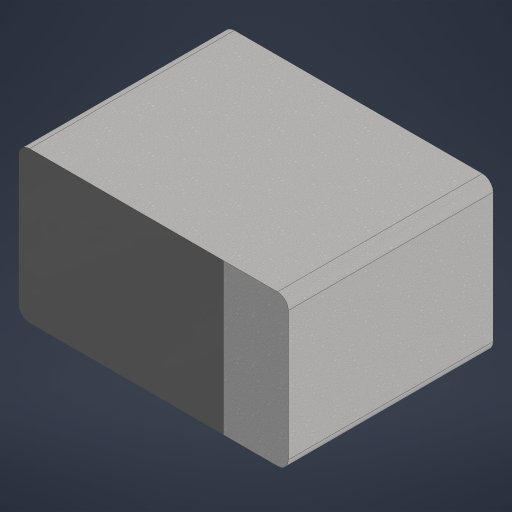
# Autodesk Inventor part: Microonde
Saved by Autodesk Inventor 2024.2 (Build 282272000, 272)
## iProperties
Created: 2025-08-13
Part Number: Microonde
Material: Steel, Galvanized
Document SubType Name: Modeling
Designer: Luca
Density: 7.85 g/cm^3
Appearance: Galvanized
Author: Luca
Autodesk Inventor part; units mm, degrees
ref_plane "YZ Plane" through (0, 0, 0) normal (1, 0, 0) x (0, 1, 0)
ref_plane "XZ Plane" through (0, 0, 0) normal (0, 1, 0) x (-1, 0, 0)
ref_plane "XY Plane" through (0, 0, 0) normal (0, 0, 1) x (1, 0, 0)
sketch "Sketch1" plane through (0, 0, 0) normal (0, 1, 0) x (-1, 0, 0)
  line L0 (250, 0) -> (-250, 0)
  line L1 (-250, 0) -> (-250, 380)
  line L2 (-250, 380) -> (250, 380)
  line L3 (250, 380) -> (250, 0)
  point P0 (0, 0)
  point P1 (0, 0)
  dimension "d0" = 500
  dimension "d1" = 380
  constraints: 8 end point, 2 parallel, 1 coincident, 1 horizontal, 1 midpoint, 1 perpendicular
  measures "d0" distance of L1.end L2.end
  measures "d1" distance of L0.end L1.end
extrude "Extrusion1" add sketch "Sketch1" along normal blind 280
fillet "Fillet1" radius 20 4 edges at (-250, 280, 190) (-250, 0, 190) (250, 0, 190) (250, 280, 190)
sketch "Sketch2" plane through (-230, 0, 380) normal (0, 0, 1) x (1, 0, 0)
  line L0 (460, 280) -> (0, 280) projected
  line L1 (360, 280) -> (360, 0)
  line L2 (480, 20) -> (480, 260) projected
  line L3 (0, 0) -> (460, 0) projected
  point P0 (230, 0)
  dimension "d5" = 120
  constraints: 2 end point, 2 point on line, 1 vertical
  measures "d5" distance between parallel lines of L2 L1
split_face "Split1"
sketch "Sketch3" plane through (0, 0, 0) normal (0, -1, 0) x (1, 0, 0)
  circle A0 centre (-190, 340) radius 15
  line L0 (230, 380) -> (230, 0) projected
  line L1 (130, 380) -> (230, 380) projected
  line L2 (-230, 380) -> (130, 380) projected
  line L3 (-230, 0) -> (-230, 380) projected
  line L4 (230, 0) -> (-230, 0) projected
  line L5 (130, 340) -> (190, 340) construction
  line L6 (190, 340) -> (190, 40) construction
  line L7 (190, 40) -> (-190, 40) construction
  line L8 (-190, 40) -> (-190, 340) construction
  line L9 (-190, 340) -> (130, 340) construction
  circle A1 centre (-190, 40) radius 15
  circle A2 centre (190, 40) radius 15
  circle A3 centre (190, 340) radius 15
  point P0 (0, 0)
  dimension "d6" = 30
  dimension "d7" = 40
  constraints: 10 end point, 4 centre point, 4 coincident, 3 equal radius, 4 other
  measures "d6" diameter of A0
  measures "d7" distance between parallel lines of L2 L9
extrude "Extrusion2" add sketch "Sketch3" along normal blind 25 contours A0 | A1 | A2 | A3
body "Solid1"
